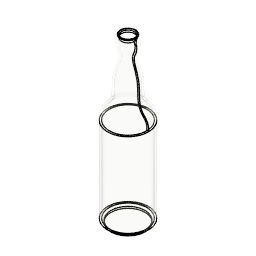
soda bottle (Autodesk Fusion 360 design; units mm, degrees)
part number: 2026-05-19-23-53-18-980
Autodesk Fusion 360 part; units mm, degrees
sketch "Sketch2" plane through (0, 0, 0) normal (0, 0, 1) x (1, 0, 0)
  line L0 (0, 0) -> (0, 240)
  line L1 (0, 0) -> (30, 0)
  line L2 (30, 0) -> (30, 130)
  spline S0 degree 5 poles (30, 130) (30.1079, 130.7828) (30.2711, 132.3079) (30.3576, 134.4733) (30.1561, 137.1162) (29.3867, 140.0223) (28.1379, 142.5665) (26.4889, 144.8219) (24.5815, 146.918) (22.606, 149.0307) (20.7587, 151.3499) (19.2115, 154.0551) (18.069, 157.2839) (17.3529, 161.1172) (17.0057, 165.5834) (16.9047, 170.6572) (16.8402, 176.2628) (16.5785, 182.2684) (15.7226, 188.4975) (14.1055, 194.6964) (12.0928, 200.5578) (10.2121, 205.8179) (9.047, 210.2949) (8.9753, 214.0249) (10.0774, 217.1915) (11.7227, 220.5349) (12.9278, 224.5448) (13.2221, 228.5743) (12.6653, 231.7954) (11.5987, 233.6066) (11.8362, 234.0462) (12.4971, 234.8332) (12.2104, 236.7496) (11.4918, 238.7895) (11, 240) knots 0 0 0 0 0 0 0.033333 0.066667 0.1 0.133333 0.166667 0.2 0.233333 0.266667 0.3 0.333333 0.366667 0.4 0.433333 0.466667 0.5 0.533333 0.566667 0.6 0.633333 0.666667 0.7 0.733333 0.766667 0.8 0.833333 0.866667 0.9 0.933333 0.966667 1 1 1 1 1 1
  line L3 (14.1411, 227.245) -> (9.8589, 238.755)
  line L4 (24, 208) -> (-2, 272)
  line L5 (6.8696, 209.0036) -> (13.7948, 226.0723)
  line L6 (17.889, 167.663) -> (14.9226, 197.5195)
  line L7 (0, 240) -> (11, 240)
  point P0 (27.3993, 143.485)
  point P1 (19.918, 152.9613)
  point P2 (16.4058, 182.5913)
  point P3 (10.3322, 217.538)
  point P4 (12, 233)
  dimension "d4" = 240
  dimension "d5" = 30
  dimension "d6" = 130
  dimension "d7" = 11
  constraint coincident L0.start L1.start
  constraint vertical L0
  constraint perpendicular L0 L1
  constraint perpendicular L1 L2
  constraint midpoint P4 L3
  constraint midpoint S0.end L4
  constraint midpoint P3 L5
  constraint midpoint P2 L6
  constraint perpendicular L0 L7
  constraint coincident S0.end L7.end
  measures "d4" distance of L0.start L0.end
  measures "d5" distance of L0.start L1.end
  measures "d6" distance of L1.end L2.end
  measures "d7" distance of L0.end S0.end
revolve "Revolve1" add sketch "Sketch2" angle 360 about axis through (0, 0, 0) along (0, 1, 0)
fillet "Fillet1" radius 5 1 edges at (-27.9698, 0, -10.8485)
shell "Shell1" thickness 2.5 removed faces 1 at (-3.2467, 240, 0.051)
fillet "Fillet2" radius 1 2 edges at (-10.2556, 240, -3.9778) (-8.3016, 240, 0.0037)
